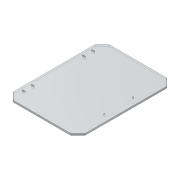
# Autodesk Inventor part: Clear Left Side Door
Saved by Autodesk Inventor 2015 (Build 190159000, 159)
## iProperties
Created: 2018-04-14
Part Number: Clear Left Side Door
Material: Glass
Document SubType Name: Modeling
Designer: Ghassan Yusuf
Density: 2.18 g/cm^3
Appearance: Clear
Author: Ghassan Yusuf
Autodesk Inventor part; units mm, degrees
ref_plane "YZ Plane" through (0, 0, 0) normal (1, 0, 0) x (0, 1, 0)
ref_plane "XZ Plane" through (0, 0, 0) normal (0, 1, 0) x (-1, 0, 0)
ref_plane "XY Plane" through (0, 0, 0) normal (0, 0, 1) x (1, 0, 0)
sketch "Handle-Hole" plane through (0, 0, 0) normal (0, 0, 1) x (1, 0, 0)
  line L0 (-99.5, 50) -> (-69.5, 50)
  line L1 (-69.5, 50) -> (-69.5, -50)
  line L2 (-69.5, -50) -> (-99.5, -50)
  line L3 (-99.5, -50) -> (-99.5, 50)
  circle A0 centre (-87.5, 62) radius 1.75
  circle A1 centre (-57.5, 27.5) radius 1.75
  circle A2 centre (-57.5, -27.5) radius 1.75
  circle A3 centre (-87.5, -62) radius 1.75
  point P0 (-82.2826, 0)
  point P1 (-99.5, 0)
  point P2 (-99.5, 0)
  dimension "d9" = 30
  dimension "d10" = 100
  dimension "d11" = 3.5
  dimension "d12" = 3.5
  dimension "d13" = 3.5
  dimension "d14" = 3.5
  dimension "d15" = 55
  dimension "d16" = 12
  dimension "d17" = 12
  dimension "d18" = 12
  measures "d9" distance of L1.end L2.end
  measures "d10" distance of L0.end L1.end
  measures "d11" diameter of A0
  measures "d12" diameter of A1
  measures "d13" diameter of A2
  measures "d14" diameter of A3
  measures "d15" distance of A2.centre A1.centre
  measures "d16" distance from line of L2 A3.centre
  measures "d17" distance from line of L0 A0.centre
  measures "d18" distance from line of L1 A1.centre
sketch "Hinges Screw Holes" plane through (0, 0, 0) normal (0, 0, 1) x (1, 0, 0)
  arc A0 (172, -72.429) -> (172, -68.929) centre (172, -70.679) ccw
  arc A1 (172, -97.929) -> (172, -94.429) centre (172, -96.179) ccw
  arc A2 (167, 97.929) -> (167, 94.429) centre (167, 96.179) ccw
  arc A3 (167, 72.429) -> (167, 68.929) centre (167, 70.679) ccw
  arc A4 (167, -68.929) -> (167, -72.429) centre (167, -70.679) ccw
  arc A5 (167, -94.429) -> (167, -97.929) centre (167, -96.179) ccw
  line L0 (167, 97.929) -> (172, 97.929)
  line L1 (167, 94.429) -> (172, 94.429)
  line L2 (167, 72.429) -> (172, 72.429)
  line L3 (167, 68.929) -> (172, 68.929)
  line L4 (167, -68.929) -> (172, -68.929)
  line L5 (167, -72.429) -> (172, -72.429)
  line L6 (167, -94.429) -> (172, -94.429)
  line L7 (167, -97.929) -> (172, -97.929)
  arc A6 (172, 94.429) -> (172, 97.929) centre (172, 96.179) ccw
  arc A7 (172, 68.929) -> (172, 72.429) centre (172, 70.679) ccw
  point P0 (169.5, 0)
  dimension "d20" = 3.5
  dimension "d26" = 141.358
  dimension "d29" = 25.5
  dimension "d31" = 3.5
  dimension "d32" = 25.5
  dimension "d34" = 5
  measures "d20" diameter of A6
  measures "d26" distance of A0.centre A7.centre
  measures "d29" distance of A3.centre A2.centre
  measures "d31" diameter of A5
  measures "d32" distance of A5.centre A4.centre
  measures "d34" distance of A6.centre A2.centre
sketch "Sketch1" plane through (0, 0, 0) normal (0, 0, 1) x (1, 0, 0)
  line L0 (-100, 133.5) -> (100, 133.5)
  line L1 (100, 133.5) -> (100, -133.5)
  line L2 (100, -133.5) -> (-100, -133.5)
  line L3 (-100, -133.5) -> (-100, 133.5)
  line L4 (99.5, 133) -> (-99.5, 133)
  line L5 (-99.5, 133) -> (-99.5, -133)
  line L6 (-99.5, -133) -> (99.5, -133)
  line L7 (99.5, -133) -> (99.5, 133)
  point P0 (0, 0)
  point P1 (0, 133.5)
  point P2 (-99.5, 0)
  dimension "d0" = 200
  dimension "d1" = 267
  dimension "d4" = 0.5
  constraints: 16 end point, 4 parallel, 2 midpoint, 2 perpendicular, 1 horizontal, 1 horizontal alignment, 1 vertical alignment, 3 other
  measures "d0" distance of L1.end L2.end
  measures "d1" distance of L0.end L1.end
  measures "d4" distance between parallel lines of L0 L4
extrude "Extrusion1" add sketch "Sketch1" along normal blind 5 contours L7 L6 L5 L4
chamfer "Chamfer1" distance 20 angle 45 4 edges at (-99.5, -133, 2.5) (-99.5, 133, 2.5) (99.5, -133, 2.5) (99.5, 133, 2.5)
fillet "Fillet1" radius 5 8 edges at (-79.5, -133, 2.5) (79.5, -133, 2.5) (99.5, -113, 2.5) (99.5, 113, 2.5) (79.5, 133, 2.5) (-79.5, 133, 2.5) (-99.5, 113, 2.5) (-99.5, -113, 2.5)
sketch "Sketch2" plane through (0, 0, 5) normal (0, 0, 1) x (1, 0, 0)
  line L0 (99.5, -110.9289) -> (99.5, 110.9289) projected
  line L1 (-99.5, 110.9289) -> (-99.5, -110.9289) projected
  circle A0 centre (79.5, 40) radius 1.75
  circle A1 centre (79.5, -40) radius 1.75
  arc A2 (-85, -72.429) -> (-85, -68.929) centre (-85, -70.679) ccw
  arc A3 (-85, -97.929) -> (-85, -94.429) centre (-85, -96.179) ccw
  arc A4 (-90, 97.929) -> (-90, 94.429) centre (-90, 96.179) ccw
  arc A5 (-90, 72.429) -> (-90, 68.929) centre (-90, 70.679) ccw
  arc A6 (-90, -68.929) -> (-90, -72.429) centre (-90, -70.679) ccw
  arc A7 (-90, -94.429) -> (-90, -97.929) centre (-90, -96.179) ccw
  line L2 (-90, 97.929) -> (-85, 97.929)
  line L3 (-90, 94.429) -> (-85, 94.429)
  line L4 (-90, 72.429) -> (-85, 72.429)
  line L5 (-90, 68.929) -> (-85, 68.929)
  line L6 (-90, -68.929) -> (-85, -68.929)
  line L7 (-90, -72.429) -> (-85, -72.429)
  line L8 (-90, -94.429) -> (-85, -94.429)
  line L9 (-90, -97.929) -> (-85, -97.929)
  arc A8 (-85, 94.429) -> (-85, 97.929) centre (-85, 96.179) ccw
  arc A9 (-85, 68.929) -> (-85, 72.429) centre (-85, 70.679) ccw
  point P0 (0, 0)
  dimension "d36" = 141.358
  dimension "d35" = 70.679
  dimension "d37" = 9.5
  dimension "d38" = 9.5
  dimension "d44" = 3.5
  dimension "d45" = 3.5
  dimension "d46" = 80
  dimension "d47" = 40
  dimension "d48" = 20
  constraints: 2 centre point, 1 vertical alignment
  measures "d44" diameter of A0
  measures "d45" diameter of A1
  measures "d46" distance of A1.centre A0.centre
  measures "d47" vertical distance of point (0, 0) A0.centre
  measures "d48" distance from line of L0 A0.centre
extrude "Extrusion2" cut sketch "Sketch2" against normal blind 10
equation "\"d35\" = 0.5 * d36"
equation "\"d47\" = 0.5 * d46"
equation "\"d16\" = d17"
equation "\"d17\" = d19"
equation "\"d18\" = d19"
equation "\"d32\" = d29"
equation "\"d19\" = 12"
body "Solid1"
